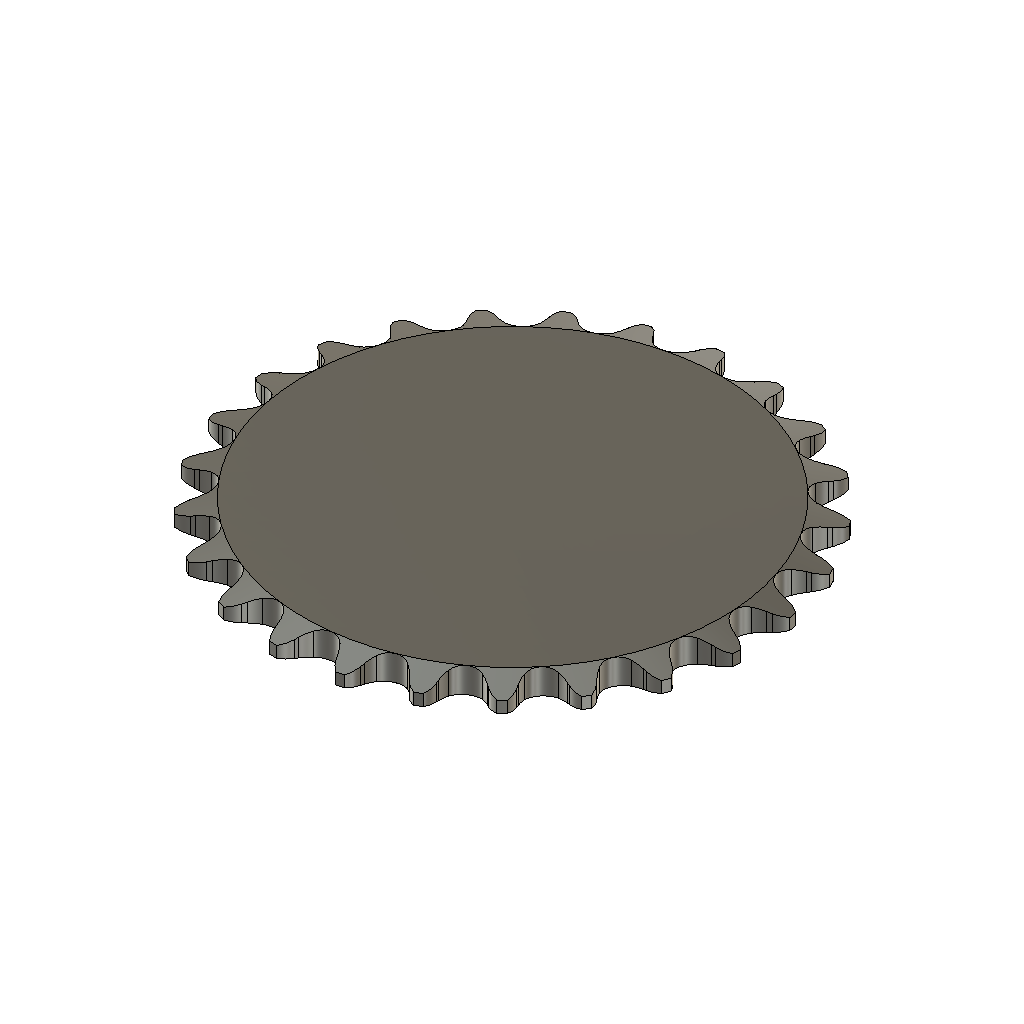
35Chain Sprocket Generator (Autodesk Fusion 360 design; units mm, degrees)
Autodesk Fusion 360 part; units mm, degrees
sketch "Teeth" plane through (0, 0, 0) normal (0, 0, 1) x (1, 0, 0)
  circle A0 centre (0, 0) radius 37.9987 construction
  line L0 (0, 37.9987) -> (-9.4499, 36.8049) construction
  arc A1 (-2.9466, 38.0172) -> (-2.0491, 36.4321) centre (3.2285, 40.4671) ccw
  line L1 (-2.9466, 38.0172) -> (-3.1936, 38.6397)
  arc A2 (-3.1936, 38.6397) -> (-4.4828, 40.3699) centre (-7.0559, 37.1073) ccw
  line L2 (0, 37.9987) -> (3.9262, 37.9987) construction
  line L3 (-2.9466, 38.0172) -> (3.2285, 40.4671) construction
  line L4 (3.2285, 40.4671) -> (0, 37.9987) construction
  line L5 (0, 37.9987) -> (0, 0) construction
  arc A3 (-2.0491, 36.4321) -> (0, 35.4193) centre (0, 37.9987) ccw
  arc A4 (4.4828, 40.3699) -> (3.1936, 38.6397) centre (7.0559, 37.1073) ccw
  line L6 (2.9466, 38.0172) -> (3.1936, 38.6397)
  arc A5 (2.0491, 36.4321) -> (2.9466, 38.0172) centre (-3.2285, 40.4671) ccw
  arc A6 (0, 35.4193) -> (2.0491, 36.4321) centre (0, 37.9987) ccw
  circle A7 centre (0, 0) radius 40.6181
  dimension "d11" = 75.9974
  dimension "d12" = 9.525
  dimension "d14" = 37.4
  dimension "d15" = 15.76
  dimension "d16" = 4.064
  dimension "d17" = 7.112
  dimension "d18" = 2.5794
  dimension "d50" = 81.2362
  constraint coincident A0.centre L5.end
  constraint coincident A0 L0.start
  constraint coincident A0 L0.end
  constraint vertical A0.centre L0.start
  constraint tangent A1 L1
  constraint tangent L1 A2
  constraint tangent A0 L2
  constraint horizontal L2
  constraint perpendicular L1 L3
  constraint coincident L0 A2.centre
  constraint coincident A1.centre L3.end
  constraint coincident L5 A3.end
  constraint coincident L0 L2.start
  constraint coincident L0.start L2.start
  constraint tangent A1 A3
  constraint symmetric A1.end L5 A5.start
  constraint symmetric A1.start L5 L6.start
  constraint symmetric A1 L5 A5
  constraint symmetric L1.end L5 A4.end
  constraint symmetric A2 L5 A4
  constraint symmetric L5 A3.end A6.start
  constraint symmetric L5 A3 A6
  constraint vertical A0.centre A3.end
  constraint coincident A2.end A7
  constraint concentric A0 A7
  constraint coincident A4.start A7
  measures "d11" diameter of A0
  measures "d12" distance of L0.start L0.end
  measures "d14" angle of L2 L4
  measures "d15" angle of L3 L4
  measures "d16" distance of A1.centre L0.start
  measures "d17" distance of A2.centre L0.start
  measures "d18" radius of A3
  measures "d50" diameter of A7
extrude "Extrude1" add sketch "Teeth" along normal mid plane 4.2926
extrude "Extrude3" cut sketch "Teeth" along normal through all and the other way through all contours A1 L1 A2 A3 A4 L6 A5 A6 A7 picked at (0.499, 38.1516)
pattern_circular "C-Pattern1" count 25 over 360 about axis through (0, 0, 0) along (0, 0, 1) of "Extrude3"
sketch "Sketch4" plane through (0, 0, 0) normal (1, 0, 0) x (0, 1, 0)
  line L0 (-40.6181, 0.9525) -> (-35.4193, 2.1463)
  line L1 (-35.4193, 2.1463) -> (0, 2.1463)
  line L2 (-7.0051, 0) -> (0, 0) construction
  line L3 (-35.4193, -2.1463) -> (0, -2.1463)
  line L4 (-40.6181, -0.9525) -> (-35.4193, -2.1463)
  line L5 (0, -2.1463) -> (0, 2.1463)
  line L6 (-40.6181, 0.9525) -> (-40.6181, -0.9525)
  point P0 (-39.6283, 3.175)
  point P1 (-40.6181, 0)
  dimension "d49" = 35.4193
  dimension "d54" = 1.905
  dimension "d55" = 4.2926
  dimension "d56" = 40.6181
  constraint coincident L2.end origin
  constraint horizontal L1
  constraint horizontal L3
  constraint midpoint L5 L2.end
  constraint perpendicular L2 L6
  constraint midpoint L6 P1
  constraint vertical L5
  constraint equal L1 L3
  constraint horizontal L2.end P1
  measures "d49" distance of L3.end L3.start
  measures "d54" distance of L0.start L4.start
  measures "d55" distance of L1.end L3.end
  measures "d56" distance of L5 L6
revolve "Revolve1" cut sketch "Sketch4" angle 360 about axis through (0, 0, 1.75) along (0, 0, 1) keep common part
equation "p = 0.375 in" comment "0.25 for #25, 0.375 for #35"
equation "Dr = 0.2 in" comment "0.13 for #25, 0.2 for #35"
equation "Ds = 1.0005 * Dr + 0.003 in"
equation "n = 25" comment "Number of Teeth"
equation "PD = p / sin(( 180 / n ) * 1 deg)"
equation "A_angle = 35 deg + ( 60 / n ) * 1 deg"
equation "B_angle = 18 deg - ( 56 / n ) * 1 deg"
equation "ac = 0.8 * Dr"
equation "ab = 1.4 * Dr"
equation "OD = PD + 0.55 * p"
equation "d11 = PD"
equation "d12 = p"
equation "d14 = A_angle"
equation "d15 = B_angle"
equation "d16 = ac"
equation "d17 = ab"
equation "d18 = Ds / 2"
equation "d49 = ( PD - Ds ) / 2"
equation "d50 = OD"
equation "d52 = n"
equation "d56 = OD / 2"
